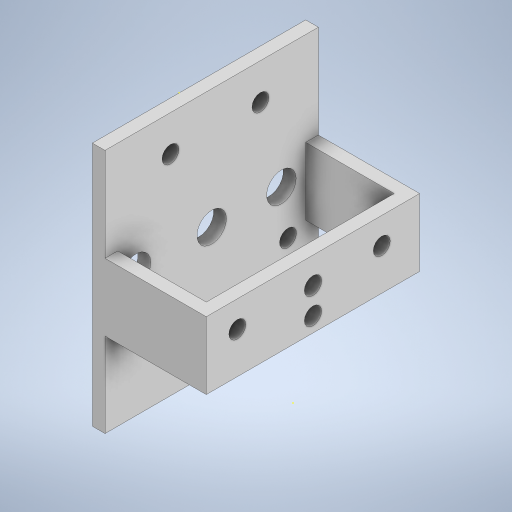
# Autodesk Inventor part: korthjulholder1
Saved by Autodesk Inventor 2023 (Build 270158000, 158)
## iProperties
Created: 2023-02-28
Part Number: korthjulholder1
Material: Generic
Document SubType Name: Modeling
Designer: Markus
Density: 1 g/cm^3
Appearance: Default
Author: Markus
Autodesk Inventor part; units mm, degrees
ref_plane "YZ Plane" through (0, 0, 0) normal (1, 0, 0) x (0, 1, 0)
ref_plane "XZ Plane" through (0, 0, 0) normal (0, 1, 0) x (-1, 0, 0)
ref_plane "XY Plane" through (0, 0, 0) normal (0, 0, 1) x (1, 0, 0)
sketch "Sketch1" plane through (0, 0, 0) normal (1, 0, 0) x (0, 1, 0)
  line L0 (0, 0) -> (20, 0)
  line L1 (20, 0) -> (20, -25)
  line L2 (20, -25) -> (0, -25)
  line L3 (0, -25) -> (0, 0)
  dimension "d0" = 20
  dimension "d1" = 25
  constraints: 8 end point, 2 parallel, 1 horizontal, 1 perpendicular
  measures "d0" distance of L1.end L2.end
  measures "d1" distance of L0.end L1.end
extrude "Extrusion1" add sketch "Sketch1" along normal blind 2
sketch "Sketch2" plane through (2, 0, 0) normal (1, 0, 0) x (0, 0, -1)
  line L0 (25, 0) -> (25, 20) projected
  line L1 (0, 0) -> (25, 0)
  line L2 (25, 0) -> (25, 2)
  line L3 (25, 2) -> (0, 2)
  line L4 (0, 2) -> (0, 0)
  dimension "d4" = 2
  constraints: 8 end point, 2 parallel, 1 horizontal, 1 perpendicular, 1 point on line
  measures "d4" distance of L2.end L1.end
extrude "Extrusion2" add sketch "Sketch2" along normal blind 25
sketch "Sketch3" plane through (2, 2, 0) normal (0, 1, 0) x (1, 0, 0)
  line L0 (-2, 0) -> (25, 0) projected
  line L1 (-2, 25) -> (25, 25) projected
  line L2 (25, 0) -> (23, 0)
  line L3 (23, 0) -> (23, 25)
  line L4 (23, 25) -> (25, 25)
  line L5 (25, 25) -> (25, 0)
  dimension "d7" = 2
  constraints: 8 end point, 2 parallel, 1 horizontal, 1 perpendicular, 1 point on line
  measures "d7" distance of L3.end L4.end
extrude "Extrusion3" add sketch "Sketch3" along normal blind 20
sketch "Sketch4" plane through (2, 0, 0) normal (1, 0, 0) x (0, 0, -1)
  point P0 (0, 0)
sketch "Sketch5" plane through (27, 0, 0) normal (1, 0, 0) x (0, 0, -1)
  circle A0 centre (6, 19.5) radius 2
  point P0 (0, 0)
  dimension "d10" = 4
  constraints: 1 centre point, 1 coincident
  measures "d10" diameter of A0
sketch "Sketch6" plane through (2, 22, 0) normal (0, 1, 0) x (1, 0, 0)
  line L0 (25, 0) -> (25, 25) projected
  line L1 (23, 25) -> (23, 0) projected
  line L2 (25, 0) -> (23, 0)
  line L3 (23, 0) -> (23, 25)
  line L4 (23, 25) -> (25, 25)
  line L5 (25, 25) -> (25, 0)
  point P0 (-2, 0)
  constraints: 8 end point, 2 parallel, 1 horizontal, 1 perpendicular
extrude "Extrusion4" add sketch "Sketch6" along normal blind 3
sketch "Sketch7" plane through (0, 20, 0) normal (0, 1, 0) x (1, 0, 0)
  line L0 (0, 25) -> (2, 25) projected
  line L1 (2, 25) -> (0, 25)
  line L2 (0, 25) -> (0, 0)
  line L3 (0, 0) -> (2, 0)
  line L4 (2, 0) -> (2, 25)
  constraints: 8 end point, 2 parallel, 1 horizontal, 1 perpendicular
extrude "Extrusion5" add sketch "Sketch7" along normal blind 5
extrude "Extrusion6" cut sketch "Sketch5" against normal blind 30
sketch "Sketch8" plane through (0, 0, 0) normal (-1, 0, 0) x (0, 0, 1)
  circle A0 centre (-22.8, 23) radius 2
  point P0 (0, 0)
  point P1 (22.8, 23)
  dimension "d17" = 4
  constraints: 1 centre point, 1 coincident
  measures "d17" diameter of A0
sketch "Sketch9" plane through (0, 0, 0) normal (-1, 0, 0) x (0, 0, 1)
  circle A0 centre (-6, 19.5) radius 2 projected
  circle A1 centre (-6, 19.5) radius 2
  point P0 (0, 0)
  constraints: 1 centre point, 1 coincident
extrude "Extrusion7" add sketch "Sketch9" against normal blind 2
extrude "Extrusion8" cut sketch "Sketch8" against normal blind 30
sketch "Sketch10" plane through (0, 0, -25) normal (-1, 0, 0) x (0, 0, 1)
  line L0 (25, 25) -> (2.2, 25) projected
  line L1 (25, 0) -> (0, 0) projected
  line L2 (12.5, 25) -> (25, 25)
  line L3 (25, 25) -> (25, 0)
  line L4 (25, 0) -> (12.5, 0)
  line L5 (12.5, 0) -> (12.5, 25)
  constraints: 8 end point, 2 parallel, 1 horizontal, 1 perpendicular, 1 point on line
extrude "Extrusion9" cut sketch "Sketch10" against normal blind 30
sketch "Sketch11" plane through (0, 0, -25) normal (-1, 0, 0) x (0, 0, 1)
  circle A0 centre (10.3, 23) radius 2
  point P0 (25, 0)
  dimension "d24" = 4
  constraints: 1 centre point, 1 coincident
  measures "d24" diameter of A0
extrude "Extrusion10" cut sketch "Sketch11" against normal blind 2.5
sketch "Sketch12" plane through (27, 0, -25) normal (1, 0, 0) x (0, 0, -1)
  circle A0 centre (-2.2, 23) radius 2 projected
  line L0 (-12.5, 25) -> (-10.3, 25) projected
  line L1 (-12.5, 2) -> (0, 2) projected
  line L2 (-12.5, 25) -> (-4.5, 25)
  line L3 (-4.5, 25) -> (-4.5, 2)
  line L4 (-4.5, 2) -> (-12.5, 2)
  line L5 (-12.5, 2) -> (-12.5, 25)
  point P0 (-25, 0)
  point P1 (-4.2, 23)
  point P2 (-2.2, 25)
  dimension "d27" = 8
  constraints: 8 end point, 2 parallel, 1 horizontal, 1 perpendicular, 1 point on circle, 1 point on line
  measures "d27" distance of L3.end L4.end
sketch "Sketch13" plane through (27, 0, -25) normal (1, 0, 0) x (0, 0, -1)
  point P0 (-25, 0)
sketch "Sketch14" plane through (0, 0, -25) normal (0, -1, 0) x (1, 0, 0)
  line L0 (27, 12.5) -> (0, 12.5) projected
  line L1 (25, 12.5) -> (25, 0) projected
  line L2 (27, 12.5) -> (25, 12.5)
  line L3 (25, 12.5) -> (25, 0)
  line L4 (25, 0) -> (27, 0)
  line L5 (27, 0) -> (27, 12.5)
  point P0 (0, 25)
  constraints: 8 end point, 2 parallel, 1 horizontal, 1 perpendicular
extrude "Extrusion11" add sketch "Sketch14" along normal blind 8
extrude "Extrusion12" cut sketch "Sketch12" against normal blind 8 contours L0 L2 L3 L1 L5
sketch "Sketch15" plane through (25, 2, -25) normal (0, 0, -1) x (-1, 0, 0)
  line L0 (0, -2) -> (0, -10) projected
  line L1 (0, -2) -> (25, -2)
  line L2 (25, -2) -> (25, 23)
  line L3 (25, 23) -> (0, 23)
  line L4 (0, 23) -> (0, -2)
  constraints: 8 end point, 2 parallel, 1 horizontal, 1 perpendicular
extrude "Extrusion13" cut sketch "Sketch15" against normal blind 30
sketch "Sketch16" plane through (27, 23, -22.8) normal (1, 0, 0) x (0, 0, -1)
  arc A0 (-0.0621, -1.999) -> (-0.0621, 1.999) centre (0, 0) ccw projected
  circle A1 centre (0, 0) radius 2
  point P0 (-22.8, -23)
  point P1 (0, 2)
  point P2 (-36, 0)
  point P3 (-0.0621, 1.999)
  point P4 (-0.0621, -1.999)
  dimension "d34" = 4
  constraints: 4 coincident, 1 centre point
  measures "d34" diameter of A1
sketch "Sketch17" plane through (25, 2, -12.5) normal (0, 0, 1) x (1, 0, 0)
  point P0 (-25, -2)
sketch "Sketch18" plane through (25, 2, -12.5) normal (0, 0, 1) x (1, 0, 0)
  line L0 (0, -10) -> (2, -10) projected
  line L1 (2, 0) -> (0, 0) projected
  line L2 (2, -10) -> (0, -10)
  line L3 (0, -10) -> (0, 0)
  line L4 (0, 0) -> (2, 0)
  line L5 (2, 0) -> (2, -10)
  point P0 (-25, -2)
  constraints: 8 end point, 2 parallel, 1 horizontal, 1 perpendicular
extrude "Extrusion14" add sketch "Sketch18" along normal blind 30
sketch "Sketch19" plane through (27, 23, -22.8) normal (1, 0, 0) x (0, 0, -1)
  point P0 (-22.8, -23)
sketch "Sketch20" plane through (25, 2, -20.5) normal (0, 1, 0) x (1, 0, 0)
  line L0 (2, 0) -> (2, 2.3) projected
  line L1 (0, 4.5) -> (0, -38) projected
  line L2 (2, 0) -> (0, 0)
  line L3 (0, 0) -> (0, -38)
  line L4 (0, -38) -> (2, -38)
  line L5 (2, -38) -> (2, 0)
  point P0 (-25, -20.5)
  constraints: 8 end point, 2 parallel, 1 horizontal, 1 perpendicular
extrude "Extrusion15" add sketch "Sketch20" along normal blind 23
sketch "Sketch21" plane through (27, 23, -22.8) normal (1, 0, 0) x (0, 0, -1)
  point P0 (-22.8, -23)
sketch "Sketch22" plane through (27, 23, -22.8) normal (1, 0, 0) x (0, 0, -1)
  point P0 (-22.8, -23)
sketch "Sketch23" plane through (27, 23, -22.8) normal (1, 0, 0) x (0, 0, -1)
  circle A0 centre (-36, 0) radius 2
  point P0 (-22.8, -23)
  dimension "d39" = 4
  constraints: 1 centre point, 1 coincident
  measures "d39" diameter of A0
extrude "Extrusion16" cut sketch "Sketch23" against normal blind 25
sketch "Sketch24" plane through (27, 23, -22.8) normal (1, 0, 0) x (0, 0, -1)
  circle A0 centre (-36, 0) radius 2 projected
  line L0 (-36, 2) -> (-40.3, 2) projected
  line L1 (2.2, -31) -> (-40.3, -31) projected
  line L2 (-40.3, 2) -> (-38.3, 2)
  line L3 (-38.3, 2) -> (-38.3, -31)
  line L4 (-38.3, -31) -> (-40.3, -31)
  line L5 (-40.3, -31) -> (-40.3, 2)
  point P0 (-22.8, -23)
  point P1 (-38, 0)
  dimension "d42" = 2
  constraints: 8 end point, 2 parallel, 1 horizontal, 1 perpendicular, 1 point on circle, 1 point on line
  measures "d42" distance of L3.end L4.end
extrude "Extrusion17" cut sketch "Sketch24" against normal blind 25 contours L3 L1 L5 L0
sketch "Sketch25" plane through (25, 23, -22.8) normal (-1, 0, 0) x (0, 0, 1)
  circle A0 centre (0, 0) radius 2 projected
  line L0 (36, 2) -> (0, 2) projected
  line L1 (2, 0) -> (2.3, 0)
  line L2 (2.3, 0) -> (2.3, 2)
  line L3 (2.3, 2) -> (2, 2)
  line L4 (2, 2) -> (2, 0)
  circle A1 centre (36, 0) radius 2 projected
  line L5 (34, 0) -> (33.7, 0)
  line L6 (33.7, 0) -> (33.7, 0.0469)
  line L7 (33.7, 0.0469) -> (34, 0.0469)
  line L8 (34, 0.0469) -> (34, 0)
  line L9 (2.3, 2) -> (33.7, 2)
  line L10 (33.7, 2) -> (33.7, 0)
  line L11 (33.7, 0) -> (2.3, 0)
  line L12 (2.3, 0) -> (2.3, 2)
  point P0 (22.8, -23)
  point P1 (2.3, 0)
  point P2 (33.7, 0.0469)
  dimension "d45" = 0.3
  dimension "d46" = 0.3
  constraints: 24 end point, 6 parallel, 3 horizontal, 3 perpendicular, 2 point on circle, 1 point on line
  measures "d45" distance of L3.end L2.end
  measures "d46" distance of L6.end L7.end
extrude "Extrusion18" cut sketch "Sketch25" against normal blind 25 contours L2 L0 L10 L6 L11
sketch "Sketch26" plane through (25, 23, -22.8) normal (-1, 0, 0) x (0, 0, 1)
  line L0 (-2.2, -31) -> (38.3, -31) projected
  line L1 (38.3, -31) -> (38.3, 2) projected
  line L2 (-2.2, -31) -> (38.3, -31)
  line L3 (38.3, -31) -> (38.3, -29)
  line L4 (38.3, -29) -> (-2.2, -29)
  line L5 (-2.2, -29) -> (-2.2, -31)
  line L6 (2.3, 0) -> (33.7, 0) projected
  line L7 (2.3, 0) -> (33.7, 0)
  line L8 (33.7, 0) -> (33.7, -29)
  line L9 (33.7, -29) -> (2.3, -29)
  line L10 (2.3, -29) -> (2.3, 0)
  point P0 (22.8, -23)
  dimension "d49" = 2
  constraints: 16 end point, 4 parallel, 2 horizontal, 2 perpendicular, 2 point on line
  measures "d49" distance of L3.end L2.end
extrude "Extrusion19" cut sketch "Sketch26" against normal blind 25 contours L10 L6 L8 L4
sketch "Sketch27" plane through (25, 23, -22.8) normal (-1, 0, 0) x (0, 0, 1)
  line L0 (-2.2, -31) -> (38.3, -31) projected
  line L1 (38.3, 2) -> (38.3, -31) projected
  line L2 (-2.2, -31) -> (38.3, -31)
  line L3 (38.3, -31) -> (38.3, -28.9821)
  line L4 (38.3, -28.9821) -> (-2.2, -28.9821)
  line L5 (-2.2, -28.9821) -> (-2.2, -31)
  point P0 (22.8, -23)
  constraints: 8 end point, 2 parallel, 1 horizontal, 1 perpendicular, 1 point on line
extrude "Extrusion20" add sketch "Sketch27" along normal blind 25
sketch "Sketch28" plane through (25, -5.9821, 10.9) normal (0, 1, 0) x (1, 0, 0)
  line L0 (2, -4.6) -> (-25, -4.6) projected
  line L1 (2, 35.9) -> (-25, 35.9) projected
  line L2 (-25, -4.6) -> (-22, -4.6)
  line L3 (-22, -4.6) -> (-22, 35.9)
  line L4 (-22, 35.9) -> (-25, 35.9)
  line L5 (-25, 35.9) -> (-25, -4.6)
  point P0 (-25, 10.9)
  dimension "d54" = 3
  constraints: 8 end point, 2 parallel, 1 horizontal, 1 perpendicular, 1 point on line
  measures "d54" distance of L4.end L3.end
extrude "Extrusion21" add sketch "Sketch28" along normal blind 31
sketch "Sketch29" plane through (27, -8, 15.5) normal (0, 0, 1) x (1, 0, 0)
  point P0 (-27, 8)
sketch "Sketch30" plane through (27, -8, 15.5) normal (0, 0, 1) x (1, 0, 0)
  line L0 (-27, 0) -> (-27, 33.0179) projected
  line L1 (-24, 2.0179) -> (-24, 33.0179) projected
  line L2 (-27, 33.0179) -> (-24, 33.0179)
  line L3 (-24, 33.0179) -> (-24, 32.9999)
  line L4 (-24, 32.9999) -> (-27, 32.9999)
  line L5 (-27, 32.9999) -> (-27, 33.0179)
  point P0 (-27, 8)
  dimension "d57" = 0.018
  constraints: 8 end point, 2 parallel, 1 horizontal, 1 perpendicular, 1 point on line
  measures "d57" distance of L2.end L3.end
extrude "Extrusion22" cut sketch "Sketch30" against normal blind 31
sketch "Sketch31" plane through (0, 23, -22.8) normal (-1, 0, 0) x (0, 0, 1)
  circle A0 centre (0, -12.5) radius 2
  point P0 (22.8, -23)
  point P1 (36, -12500)
  point P2 (36, -12500)
  dimension "d60" = 4
  constraints: 2 coincident, 1 centre point
  measures "d60" diameter of A0
sketch "Sketch32" plane through (0, 23, -22.8) normal (-1, 0, 0) x (0, 0, 1)
  circle A0 centre (36.1, -12.4998) radius 2
  point P0 (22.8, -23)
  point P1 (-0.0002, -12.4998)
  dimension "d61" = 4
  constraints: 1 centre point, 1 coincident
  measures "d61" diameter of A0
extrude "Extrusion23" cut sketch "Sketch31" against normal blind 3
extrude "Extrusion24" cut sketch "Sketch32" against normal blind 3
fillet "Fillet1" radius 2 2 edges at (1.5, 24.9999, 15.5) (1.5, 25.0179, -25)
fillet "Fillet2" radius 2 2 edges at (0, -8, -4.75) (27, -8, -4.75)
sketch "Sketch33" plane through (0, 23, -22.8) normal (-1, 0, 0) x (0, 0, 1)
  point P0 (22.8, -23)
sketch "Sketch34" plane through (0, 23, -22.8) normal (-1, 0, 0) x (0, 0, 1)
  circle A0 centre (18.05, -4) radius 2
  point P0 (22.8, -23)
  dimension "d68" = 4
  constraints: 1 centre point, 1 coincident
  measures "d68" diameter of A0
extrude "Extrusion25" cut sketch "Sketch34" against normal blind 3
sketch "Sketch35" plane through (27, 23, 13.2) normal (1, 0, 0) x (0, 0, -1)
  point P0 (13.2, -23)
sketch "Sketch36" plane through (25, -6, 10.9) normal (0, 1, 0) x (1, 0, 0)
  line L0 (0, 0) -> (2, 0) projected
  line L1 (0, 0) -> (0, 31.4) projected
  line L2 (2, 0) -> (0, 0)
  line L3 (0, 0) -> (0, 31.4)
  line L4 (0, 31.4) -> (2, 31.4)
  line L5 (2, 31.4) -> (2, 0)
  point P0 (-25, 10.9)
  constraints: 8 end point, 2 parallel, 1 horizontal, 1 perpendicular
extrude "Extrusion26" add sketch "Sketch36" along normal blind 3
sketch "Sketch37" plane through (27, 23, -22.8) normal (1, 0, 0) x (0, 0, -1)
  point P0 (-22.8, -23)
sketch "Sketch38" plane through (25, -3, 10.9) normal (0, 1, 0) x (1, 0, 0)
  line L0 (2, 0) -> (0, 0) projected
  line L1 (2, 35.9) -> (2, -4.6) projected
  line L2 (0, 0) -> (2, 0)
  line L3 (2, 0) -> (2, 31.4499)
  line L4 (2, 31.4499) -> (0, 31.4499)
  line L5 (0, 31.4499) -> (0, 0)
  point P0 (-25, 10.9)
  constraints: 8 end point, 2 parallel, 1 horizontal, 1 perpendicular, 1 point on line
extrude "Extrusion27" add sketch "Sketch38" along normal blind 3
sketch "Sketch39" plane through (25, 0, 10.9) normal (0, 1, 0) x (1, 0, 0)
  line L0 (0, 31.4) -> (0, 0) projected
  line L1 (2, 0) -> (2, 31.4) projected
  line L2 (0, 0) -> (2, 0)
  line L3 (2, 0) -> (2, 31.4)
  line L4 (2, 31.4) -> (0, 31.4)
  line L5 (0, 31.4) -> (0, 0)
  point P0 (-25, 10.9)
  constraints: 8 end point, 2 parallel, 1 horizontal, 1 perpendicular
extrude "Extrusion28" add sketch "Sketch39" along normal blind 25
sketch "Sketch40" plane through (27, 23, -22.8) normal (1, 0, 0) x (0, 0, -1)
  point P0 (-22.8, -23)
sketch "Sketch41" plane through (2, 25, 0) normal (0, 1, 0) x (1, 0, 0)
  line L0 (25, -15.5) -> (23, -15.5) projected
  line L1 (25, 22.8) -> (25, 25) projected
  line L2 (23, -15.5) -> (25, -15.5)
  line L3 (25, -15.5) -> (25, 25)
  line L4 (25, 25) -> (23, 25)
  line L5 (23, 25) -> (23, -15.5)
  point P0 (-2, 0)
  constraints: 8 end point, 2 parallel, 1 horizontal, 1 perpendicular
extrude "Extrusion29" add sketch "Sketch41" along normal blind 3
sketch "Sketch42" plane through (3, -5.9821, 15.5) normal (0, 0, 1) x (1, 0, 0)
  line L0 (22, 0) -> (0, 0) projected
  line L1 (24, 33.9821) -> (24, -0.0179) projected
  line L2 (22, 0) -> (24, 0)
  line L3 (24, 0) -> (24, 33.9821)
  line L4 (24, 33.9821) -> (22, 33.9821)
  line L5 (22, 33.9821) -> (22, 0)
  point P0 (-3, 5.9821)
  constraints: 8 end point, 2 parallel, 1 horizontal, 1 perpendicular
extrude "Extrusion30" add sketch "Sketch42" along normal blind 5
sketch "Sketch43" plane through (25, -5.9821, -25) normal (0, 0, -1) x (-1, 0, 0)
  arc A0 (-2, -0.0179) -> (0, -2.0179) centre (0, -0.0179) ccw projected
  line L0 (0, 33.9821) -> (0, 0) projected
  line L1 (-2, -0.0179) -> (0, -0.0179)
  line L2 (0, -0.0179) -> (0, 33.9821)
  line L3 (0, 33.9821) -> (-2, 33.9821)
  line L4 (-2, 33.9821) -> (-2, -0.0179)
  point P0 (25, 5.9821)
  constraints: 8 end point, 2 parallel, 1 horizontal, 1 perpendicular
extrude "Extrusion31" add sketch "Sketch43" along normal blind 5
sketch "Sketch44" plane through (25, -5.9821, -25) normal (0, 0, -1) x (-1, 0, 0)
  point P0 (25, 5.9821)
sketch "Sketch45" plane through (0, -8, -25) normal (0, -1, 0) x (1, 0, 0)
  point P0 (0, 25)
sketch "Sketch46" plane through (0, -8, -25) normal (0, -1, 0) x (1, 0, 0)
  line L0 (27, 40.5) -> (0, 40.5)
  line L1 (0, 40.5) -> (0, 0)
  line L2 (0, 0) -> (27, 0)
  line L3 (27, 0) -> (27, 40.5)
  point P0 (0, 25)
  constraints: 8 end point, 2 parallel, 1 horizontal, 1 perpendicular
extrude "Extrusion32" cut sketch "Sketch46" against normal up to surface (2.0179 mm away)
sketch "Sketch47" plane through (27, 0, 0) normal (1, 0, 0) x (0, 0, -1)
  point P0 (0, 0)
sketch "Sketch48" plane through (25, -5.9821, 20.5) normal (0, -1, 0) x (1, 0, 0)
  line L0 (2, -50.5) -> (0, -50.5) projected
  line L1 (2, -50.5) -> (-25, -50.5)
  line L2 (-25, -50.5) -> (-25, 0.0671)
  line L3 (-25, 0.0671) -> (2, 0.0671)
  line L4 (2, 0.0671) -> (2, -50.5)
  point P0 (-25, -20.5)
  constraints: 8 end point, 2 parallel, 1 horizontal, 1 perpendicular
extrude "Extrusion33" add sketch "Sketch48" along normal blind 2
sketch "Sketch49" plane through (0, 23, -22.8) normal (-1, 0, 0) x (0, 0, 1)
  line L0 (-2.2, -28.9821) -> (-2.2, 0.0179) projected
  line L1 (-2.2, 0.0179) -> (38.3, 0.0179)
  line L2 (38.3, 0.0179) -> (38.3, 1.9999)
  line L3 (38.3, 1.9999) -> (-2.2, 1.9999)
  line L4 (-2.2, 1.9999) -> (-2.2, 0.0179)
  point P0 (22.8, -23)
  constraints: 8 end point, 2 parallel, 1 horizontal, 1 perpendicular
extrude "Extrusion34" cut sketch "Sketch49" against normal blind 5
sketch "Sketch50" plane through (0, 23, -22.8) normal (-1, 0, 0) x (0, 0, 1)
  line L0 (7.3, 1.9999) -> (-0.4677, 1.9999) projected
  line L1 (-0.4677, 1.9999) -> (7.3, 1.9999)
  line L2 (7.3, 1.9999) -> (7.3, 2.0583)
  line L3 (7.3, 2.0583) -> (-0.4677, 2.0583)
  line L4 (-0.4677, 2.0583) -> (-0.4677, 1.9999)
  point P0 (22.8, -23)
  constraints: 8 end point, 2 parallel, 1 horizontal, 1 perpendicular
extrude "Extrusion35" cut sketch "Sketch50" against normal blind 5
sketch "Sketch51" plane through (25, -5.9821, 20.5) normal (0, 1, 0) x (1, 0, 0)
  line L0 (-25, 45.5) -> (-25, 50.5) projected
  line L1 (-22, 45.5) -> (-25, 45.5) projected
  line L2 (-25, 50.5) -> (-22, 50.5)
  line L3 (-22, 50.5) -> (-22, 45.5)
  line L4 (-22, 45.5) -> (-25, 45.5)
  line L5 (-25, 45.5) -> (-25, 50.5)
  line L6 (-25, 5) -> (-22, 5) projected
  line L7 (-25, -0.0671) -> (-25, 5) projected
  line L8 (-22, 5) -> (-25, 5)
  line L9 (-25, 5) -> (-25, -0.0671)
  line L10 (-25, -0.0671) -> (-22, -0.0671)
  line L11 (-22, -0.0671) -> (-22, 5)
  point P0 (-25, 20.5)
  constraints: 16 end point, 4 parallel, 2 horizontal, 2 perpendicular
extrude "Extrusion36" add sketch "Sketch51" along normal up to surface (29 mm away)
sketch "Sketch52" plane through (0, 23.0179, 15.4999) normal (0, 1, 0) x (1, 0, 0)
  line L0 (3, 0) -> (3, 45.4999) projected
  line L1 (0, -0.0001) -> (0, -5.0672) projected
  line L2 (3, 45.4999) -> (0, 45.4999)
  line L3 (0, 45.4999) -> (0, -5.0672)
  line L4 (0, -5.0672) -> (3, -5.0672)
  line L5 (3, -5.0672) -> (3, 45.4999)
  point P0 (0, 15.4999)
  constraints: 8 end point, 2 parallel, 1 horizontal, 1 perpendicular
extrude "Extrusion37" add sketch "Sketch52" along normal blind 50
sketch "Sketch53" plane through (0, 23, -22.8) normal (-1, 0, 0) x (0, 0, 1)
  circle A0 centre (18.05, -4) radius 2 projected
  circle A1 centre (0, -12.5) radius 2 projected
  circle A2 centre (36.1, -12.4998) radius 2 projected
  circle A3 centre (0, 38.0418) radius 2
  circle A4 centre (18.05, 38.0418) radius 2
  circle A5 centre (36.1, 38.0418) radius 2
  circle A6 centre (18.05, -4) radius 2
  point P0 (22.8, -23)
  dimension "d95" = 4
  dimension "d96" = 4
  dimension "d97" = 4
  constraints: 7 coincident, 4 centre point, 1 concentric
  measures "d95" diameter of A3
  measures "d96" diameter of A4
  measures "d97" diameter of A5
extrude "Extrusion38" cut sketch "Sketch53" against normal blind 50 contours A3 | A4 | A5
sketch "Sketch54" plane through (0, 23, -22.8) normal (-1, 0, 0) x (0, 0, 1)
  circle A0 centre (18.05, -4) radius 2 projected
  circle A1 centre (18.05, -4) radius 2
  point P0 (22.8, -23)
  constraints: 2 coincident, 1 centre point, 1 concentric
extrude "Extrusion39" add sketch "Sketch54" against normal blind 3
sketch "Sketch55" plane through (25, -5.9821, 20.5) normal (0, 1, 0) x (1, 0, 0)
  line L0 (0, 50.5) -> (2, 50.5) projected
  line L1 (2, -0.0671) -> (-22, -0.0671) projected
  line L2 (0, 50.5) -> (-1, 50.5)
  line L3 (-1, 50.5) -> (-1, -0.0671)
  line L4 (-1, -0.0671) -> (0, -0.0671)
  line L5 (0, -0.0671) -> (0, 50.5)
  point P0 (-25, 20.5)
  point P1 (0, -0.0671)
  dimension "d102" = 1
  constraints: 8 end point, 2 parallel, 1 horizontal, 1 perpendicular, 1 point on line
  measures "d102" distance of L4.end L3.end
extrude "Extrusion40" add sketch "Sketch55" along normal up to surface (33.9821 mm away)
sketch "Sketch56" plane through (25, -5.9821, 20.5) normal (0, 1, 0) x (1, 0, 0)
  line L0 (-22, 50.5) -> (-1, 50.5) projected
  line L1 (0, -0.0671) -> (-1, -0.0671) projected
  line L2 (-22, 50.5) -> (-1, 50.5)
  line L3 (-1, 50.5) -> (-1, -0.0671)
  line L4 (-1, -0.0671) -> (-22, -0.0671)
  line L5 (-22, -0.0671) -> (-22, 50.5)
  point P0 (-25, 20.5)
  constraints: 8 end point, 2 parallel, 1 horizontal, 1 perpendicular
extrude "Extrusion41" add sketch "Sketch56" along normal blind 1
sketch "Sketch57" plane through (3, -5.9821, 20.5) normal (0, 0, 1) x (1, 0, 0)
  line L0 (22, 0) -> (22, 33.9821) projected
  line L1 (24, 33.9821) -> (24, -2) projected
  line L2 (22, 33.9821) -> (24, 33.9821)
  line L3 (24, 33.9821) -> (24, -0.0257)
  line L4 (24, -0.0257) -> (22, -0.0257)
  line L5 (22, -0.0257) -> (22, 33.9821)
  point P0 (-3, 5.9821)
  constraints: 8 end point, 2 parallel, 1 horizontal, 1 perpendicular, 1 point on line
extrude "Extrusion42" add sketch "Sketch57" along normal up to surface (0.0671 mm away)
sketch "Sketch58" plane through (27, 0, 0) normal (1, 0, 0) x (0, 0, -1)
  point P0 (0, 0)
sketch "Sketch59" plane through (25, 23, 13.2) normal (1, 0, 0) x (0, 0, -1)
  circle A0 centre (0, 0) radius 1.9931
  circle A1 centre (36.0442, 0) radius 2.0019
  point P0 (13.2, -23)
  constraints: 2 centre point, 1 coincident
extrude "Extrusion43" cut sketch "Sketch59" against normal blind 10
sketch "Sketch60" plane through (27, 0, 0) normal (1, 0, 0) x (0, 0, -1)
  circle A0 centre (4.75, 61.0418) radius 2 projected
  line L0 (-1.2836, 17.728) -> (10.7164, 17.728)
  line L1 (10.7164, 17.728) -> (10.7164, 28)
  line L2 (10.7164, 28) -> (-1.2836, 28)
  line L3 (-1.2836, 28) -> (-1.2836, 17.728)
  line L4 (-1.2836, 17.728) -> (10.7164, 28) construction
  line L5 (10.7164, 17.728) -> (-1.2836, 28) construction
  line L6 (-1.2836, 22.864) -> (10.7164, 22.864)
  line L7 (10.7164, 22.864) -> (10.7164, 28)
  line L8 (10.7164, 28) -> (-1.2836, 28)
  line L9 (-1.2836, 28) -> (-1.2836, 22.864)
  point P0 (0, 0)
  point P1 (4.7164, 22.864)
  dimension "d111" = 12
  constraints: 20 end point, 4 parallel, 3 midpoint, 2 horizontal, 2 perpendicular, 1 coincident
  measures "d111" distance of L0.start L0.end
extrude "Extrusion44" cut sketch "Sketch60" against normal blind 10 contours L3 L2 L1 L6
fillet "Fillet3" radius 2 2 edges at (25.5, 28, 1.2836) (25.5, 28, -10.7164)
sketch "Sketch61" plane through (27, 0, 0) normal (1, 0, 0) x (0, 0, -1)
  line L0 (-1.2836, 22.864) -> (10.7164, 22.864)
  line L1 (10.7164, 22.864) -> (10.7164, 18.864)
  line L2 (10.7164, 18.864) -> (-1.2836, 18.864)
  line L3 (-1.2836, 18.864) -> (-1.2836, 22.864)
  point P0 (0, 0)
  dimension "d115" = 4
  constraints: 8 end point, 2 parallel, 1 horizontal, 1 perpendicular
  measures "d115" distance of L0.end L1.end
extrude "Extrusion45" cut sketch "Sketch61" against normal blind 10
sketch "Sketch62" plane through (25, -7.9821, 20.5) normal (0, -1, 0) x (1, 0, 0)
  point P0 (-25, -20.5)
sketch "Sketch63" plane through (27, 0, 0) normal (1, 0, 0) x (0, 0, -1)
  line L0 (-1.2836, 18.864) -> (10.7164, 18.864) projected
  line L1 (12.7164, 28) -> (30, 28) projected
  line L2 (10.7164, 18.864) -> (16.2164, 18.864)
  line L3 (16.2164, 18.864) -> (16.2164, 28)
  line L4 (16.2164, 28) -> (10.7164, 28)
  line L5 (10.7164, 28) -> (10.7164, 18.864)
  line L6 (-1.2836, 26) -> (-1.2836, 18.864) projected
  line L7 (-20.5671, 28) -> (-3.2836, 28) projected
  line L8 (-1.2836, 18.864) -> (-6.7836, 18.864)
  line L9 (-6.7836, 18.864) -> (-6.7836, 28)
  line L10 (-6.7836, 28) -> (-1.2836, 28)
  line L11 (-1.2836, 28) -> (-1.2836, 18.864)
  point P0 (0, 0)
  dimension "d118" = 5.5
  dimension "d119" = 5.5
  constraints: 16 end point, 4 parallel, 2 horizontal, 2 perpendicular, 2 point on line
  measures "d118" distance of L4.end L3.end
  measures "d119" distance of L9.end L10.end
extrude "Extrusion46" cut sketch "Sketch63" against normal blind 10
sketch "Sketch64" plane through (25, -4.9821, 20.5) normal (0, 1, 0) x (1, 0, 0)
  line L0 (-25, -0.0671) -> (-22, -0.0671) projected
  line L1 (-1, 50.5) -> (-1, -0.0671) projected
  line L2 (-22, -0.0671) -> (-1, -0.0671)
  line L3 (-1, -0.0671) -> (-1, 2.9329)
  line L4 (-1, 2.9329) -> (-22, 2.9329)
  line L5 (-22, 2.9329) -> (-22, -0.0671)
  line L6 (-1, 50.5) -> (-22, 50.5) projected
  line L7 (-22, 50.5) -> (-1, 50.5)
  line L8 (-1, 50.5) -> (-1, 47.5)
  line L9 (-1, 47.5) -> (-22, 47.5)
  line L10 (-22, 47.5) -> (-22, 50.5)
  point P0 (-25, 20.5)
  point P1 (-1, 47.5)
  dimension "d122" = 3
  dimension "d123" = 3
  constraints: 16 end point, 4 parallel, 2 horizontal, 2 perpendicular, 2 point on line
  measures "d122" distance of L3.end L2.end
  measures "d123" distance of L7.end L8.end
extrude "Extrusion47" add sketch "Sketch64" along normal up to surface (32.9821 mm away)
sketch "Sketch65" plane through (0, -7.9821, 20.5671) normal (0, 0, 1) x (1, 0, 0)
  line L0 (3, 3) -> (24, 3) projected
  line L1 (24, 3) -> (24, 35.9821) projected
  line L2 (3, 3) -> (24, 3)
  line L3 (24, 3) -> (24, 9.5)
  line L4 (24, 9.5) -> (3, 9.5)
  line L5 (3, 9.5) -> (3, 3)
  point P0 (0, 7.9821)
  dimension "d126" = 6.5
  constraints: 8 end point, 2 parallel, 1 horizontal, 1 perpendicular, 1 point on line
  measures "d126" distance of L3.end L2.end
extrude "Extrusion48" cut sketch "Sketch65" against normal blind 70
fillet "Fillet4" radius 2 2 edges at (25.5, 28, 6.7836) (25.5, 28, -16.2164)
fillet "Fillet5" radius 2 2 edges at (1.5, 73.0179, -30) (1.5, 73.0179, 20.5671)
sketch "Sketch66" plane through (27, 0, 0) normal (1, 0, 0) x (0, 0, -1)
  line L0 (-8.7836, 28) -> (18.2164, 28)
  line L1 (18.2164, 28) -> (18.2164, 15.9597)
  line L2 (18.2164, 15.9597) -> (-8.7836, 15.9597)
  line L3 (-8.7836, 15.9597) -> (-8.7836, 28)
  point P0 (0, 0)
  constraints: 8 end point, 2 parallel, 1 horizontal, 1 perpendicular
extrude "Extrusion49" cut sketch "Sketch66" against normal blind 10
sketch "Sketch67" plane through (27, 0, 0) normal (1, 0, 0) x (0, 0, -1)
  point P0 (0, 0)
sketch "Sketch68" plane through (27, 0, 0) normal (1, 0, 0) x (0, 0, -1)
  point P0 (0, 0)
sketch "Sketch69" plane through (27, 0, 0) normal (1, 0, 0) x (0, 0, -1)
  point P0 (0, 0)
fillet "Fillet6" radius 2 2 edges at (25.5, 28, 8.7836) (25.5, 28, -18.2164)
sketch "Sketch70" plane through (0, 23, -22.8) normal (-1, 0, 0) x (0, 0, 1)
  line L0 (-7.2, 50.0179) -> (43.5303, 50.0179)
  line L1 (43.5303, 50.0179) -> (43.5303, 46.0179)
  line L2 (43.5303, 46.0179) -> (-7.2, 46.0179)
  line L3 (-7.2, 46.0179) -> (-7.2, 50.0179)
  point P0 (22.8, -23)
  dimension "d134" = 4
  constraints: 8 end point, 2 parallel, 1 horizontal, 1 perpendicular
  measures "d134" distance of L0.end L1.end
extrude "Extrusion50" add sketch "Sketch70" along normal blind 19
sketch "Sketch71" plane through (-19, 23, -22.8) normal (-1, 0, 0) x (0, 0, 1)
  line L0 (-5.2, 50.0179) -> (-7.2, 50.0179) projected
  line L1 (43.3671, 48.0179) -> (43.3671, 46.0179) projected
  line L2 (-7.2, 50.0179) -> (43.3671, 50.0179)
  line L3 (43.3671, 50.0179) -> (43.3671, 46.0179)
  line L4 (43.3671, 46.0179) -> (-7.2, 46.0179)
  line L5 (-7.2, 46.0179) -> (-7.2, 50.0179)
  point P0 (22.8, -23)
  constraints: 8 end point, 2 parallel, 1 horizontal, 1 perpendicular
extrude "Extrusion51" add sketch "Sketch71" along normal blind 3
sketch "Sketch72" plane through (0, 69.0179, -30) normal (0, -1, 0) x (1, 0, 0)
  line L0 (-19, 50.5671) -> (-22, 50.5671) projected
  line L1 (0, 0) -> (-22, 0) projected
  line L2 (-22, 50.5671) -> (-18.2142, 50.5671)
  line L3 (-18.2142, 50.5671) -> (-18.2142, 0)
  line L4 (-18.2142, 0) -> (-22, 0)
  line L5 (-22, 0) -> (-22, 50.5671)
  point P0 (0, 30)
  constraints: 8 end point, 2 parallel, 1 horizontal, 1 perpendicular, 1 point on line
extrude "Extrusion52" add sketch "Sketch72" along normal blind 20
fillet "Fillet7" radius 2 5 edges at (-9.5, 73.0179, 20.7303) (-11, 73.0179, -30) (-22, 73.0179, -4.7164) (-22, 61.0179, 20.5671) (-22, 61.0179, -30)
sketch "Sketch73" plane through (3, -4.9821, 20.5671) normal (1, 0, 0) x (0, 0, -1)
  line L0 (0, 74) -> (0, -3) projected
  line L1 (50.5671, 54) -> (0, 54) projected
  line L2 (0, 33.122) -> (50.5671, 33.122)
  line L3 (50.5671, 33.122) -> (50.5671, 54)
  line L4 (50.5671, 54) -> (0, 54)
  line L5 (0, 54) -> (0, 33.122)
  point P0 (20.5671, 4.9821)
  constraints: 8 end point, 2 parallel, 1 horizontal, 1 perpendicular, 1 point on line
extrude "Extrusion53" cut sketch "Sketch73" against normal blind 10
sketch "Sketch74" plane through (3, 73.0179, 18.5671) normal (1, 0, 0) x (0, 0, -1)
  point P0 (18.5671, -73.0179)
sketch "Sketch75" plane through (3, 73.0179, 18.5671) normal (1, 0, 0) x (0, 0, -1)
  line L0 (48.5671, -24) -> (-2, -24) projected
  line L1 (-2, -24) -> (48.5671, -24)
  line L2 (48.5671, -24) -> (48.5671, 2.4368)
  line L3 (48.5671, 2.4368) -> (-2, 2.4368)
  line L4 (-2, 2.4368) -> (-2, -24)
  point P0 (18.5671, -73.0179)
  constraints: 8 end point, 2 parallel, 1 horizontal, 1 perpendicular
extrude "Extrusion54" cut sketch "Sketch75" against normal blind 40
sketch "Sketch76" plane through (-19, 69.0179, 20.7303) normal (0, 0, 1) x (1, 0, 0)
  line L0 (-12.4602, -22.1181) -> (25.8897, -22.1181)
  line L1 (25.8897, -22.1181) -> (25.8897, 34.1617)
  line L2 (25.8897, 34.1617) -> (-12.4602, 34.1617)
  line L3 (-12.4602, 34.1617) -> (-12.4602, -22.1181)
  point P0 (19, -69.0179)
  constraints: 8 end point, 2 parallel, 1 horizontal, 1 perpendicular
extrude "Extrusion55" cut sketch "Sketch76" against normal blind 40
sketch "Sketch77" plane through (3, 28.1399, 20.5671) normal (0, 1, 0) x (1, 0, 0)
  line L0 (-3, 0) -> (-3, 50.5671) projected
  line L1 (0, 0) -> (0, 3) projected
  line L2 (-3, 50.5671) -> (0, 50.5671)
  line L3 (0, 50.5671) -> (0, 0)
  line L4 (0, 0) -> (-3, 0)
  line L5 (-3, 0) -> (-3, 50.5671)
  point P0 (-3, 20.5671)
  constraints: 8 end point, 2 parallel, 1 horizontal, 1 perpendicular
extrude "Extrusion56" add sketch "Sketch77" along normal blind 22
sketch "Sketch78" plane through (0, 23, -22.8) normal (-1, 0, 0) x (0, 0, 1)
  line L0 (43.3671, 27.1399) -> (-7.2, 27.1399) projected
  line L1 (-7.2, 27.1399) -> (44.6312, 27.1399)
  line L2 (44.6312, 27.1399) -> (44.6312, 24.1399)
  line L3 (44.6312, 24.1399) -> (-7.2, 24.1399)
  line L4 (-7.2, 24.1399) -> (-7.2, 27.1399)
  point P0 (22.8, -23)
  dimension "d150" = 3
  constraints: 8 end point, 2 parallel, 1 horizontal, 1 perpendicular
  measures "d150" distance of L1.end L2.end
extrude "Extrusion57" add sketch "Sketch78" along normal blind 21
sketch "Sketch79" plane through (0, 47.1399, -30) normal (0, -1, 0) x (1, 0, 0)
  line L0 (0, 0) -> (-21, 0) projected
  line L1 (0, 51.8312) -> (-21, 51.8312) projected
  line L2 (-21, 0) -> (-18, 0)
  line L3 (-18, 0) -> (-18, 51.8312)
  line L4 (-18, 51.8312) -> (-21, 51.8312)
  line L5 (-21, 51.8312) -> (-21, 0)
  point P0 (0, 30)
  dimension "d153" = 3
  constraints: 8 end point, 2 parallel, 1 horizontal, 1 perpendicular, 1 point on line
  measures "d153" distance of L4.end L3.end
extrude "Extrusion58" add sketch "Sketch79" along normal blind 21
sketch "Sketch80" plane through (0, 47.1399, 21.8312) normal (0, 0, 1) x (1, 0, 0)
  line L0 (-21, 3) -> (-21, -21) projected
  line L1 (3, 3) -> (-21, 3) projected
  line L2 (-21, -21) -> (0, -21)
  line L3 (0, -21) -> (0, 3)
  line L4 (0, 3) -> (-21, 3)
  line L5 (-21, 3) -> (-21, -21)
  point P0 (0, -47.1399)
  constraints: 8 end point, 2 parallel, 1 horizontal, 1 perpendicular, 1 point on line
extrude "Extrusion59" cut sketch "Sketch80" against normal up to surface (1.2641 mm away)
sketch "Sketch81" plane through (-21, 23, -22.8) normal (-1, 0, 0) x (0, 0, 1)
  circle A0 centre (36.1, -12.4998) radius 2 projected
  circle A1 centre (0.0369, 9.7943) radius 2
  circle A2 centre (36.1, 9.7943) radius 2
  point P0 (22.8, -23)
  dimension "d158" = 4
  dimension "d159" = 4
  constraints: 3 coincident, 2 centre point
  measures "d158" diameter of A1
  measures "d159" diameter of A2
extrude "Extrusion60" cut sketch "Sketch81" against normal blind 4 contours A1 | A2
sketch "Sketch82" plane through (-21, 23, -22.8) normal (-1, 0, 0) x (0, 0, 1)
  circle A0 centre (18.0836, 17.9735) radius 2
  point P0 (22.8, -23)
  dimension "d162" = 4
  constraints: 1 centre point
  measures "d162" diameter of A0
extrude "Extrusion61" cut sketch "Sketch82" against normal blind 4
sketch "Sketch83" plane through (27, 0, 0) normal (1, 0, 0) x (0, 0, -1)
  line L0 (-20.5671, 28) -> (-20.5671, -7.9821) projected
  line L1 (30, 28) -> (30, -7.9821) projected
  line L2 (-20.5671, 28) -> (30, 28)
  line L3 (30, 28) -> (30, 15.653)
  line L4 (30, 15.653) -> (-20.5671, 15.653)
  line L5 (-20.5671, 15.653) -> (-20.5671, 28)
  point P0 (0, 0)
  constraints: 8 end point, 2 parallel, 1 horizontal, 1 perpendicular, 1 point on line
extrude "Extrusion62" cut sketch "Sketch83" against normal up to surface (3 mm away)
sketch "Sketch84" plane through (27, 15.653, 20.5671) normal (0, 1, 0) x (1, 0, 0)
  line L0 (0, 50.5671) -> (0, 0) projected
  line L1 (-3, 0) -> (-3, 50.5671) projected
  line L2 (0, 50.5671) -> (-3, 50.5671)
  line L3 (-3, 50.5671) -> (-3, 0)
  line L4 (-3, 0) -> (0, 0)
  line L5 (0, 0) -> (0, 50.5671)
  point P0 (-27, 20.5671)
  constraints: 8 end point, 2 parallel, 1 horizontal, 1 perpendicular
extrude "Extrusion63" add sketch "Sketch84" along normal up to surface (12.347 mm away)
sketch "Sketch85" plane through (3, 50.1399, 20.5671) normal (0, 1, 0) x (1, 0, 0)
  point P0 (-3, 20.5671)
sketch "Sketch86" plane through (27, 0, 0) normal (1, 0, 0) x (0, 0, -1)
  line L0 (30, -7.9821) -> (-20.5671, -7.9821) projected
  circle A0 centre (4.7164, 21.7437) radius 2.05
  point P0 (0, 0)
  point P1 (4.7164, -7.9821)
  point P2 (-13.3386, 21.7437)
  point P3 (18.8202, 21.7437)
  dimension "d169" = 4.1
  constraints: 1 centre point, 1 coincident, 1 midpoint
  measures "d169" diameter of A0
extrude "Extrusion64" cut sketch "Sketch86" against normal blind 50
sketch "Sketch87" plane through (27, 0, 0) normal (1, 0, 0) x (0, 0, -1)
  circle A0 centre (4.7164, 21.7437) radius 2.05 projected
  circle A1 centre (-13.2168, 21.7437) radius 2
  circle A2 centre (21.0128, 21.7437) radius 2
  point P0 (0, 0)
  dimension "d172" = 4
  dimension "d173" = 4
  constraints: 3 coincident, 2 centre point
  measures "d172" diameter of A1
  measures "d173" diameter of A2
extrude "Extrusion65" cut sketch "Sketch87" against normal blind 50 contours A1 | A2
sketch "Sketch88" plane through (0, 23, -22.8) normal (-1, 0, 0) x (0, 0, 1)
  circle A0 centre (18.0836, -1.2563) radius 2.05 projected
  circle A1 centre (18.0836, -1.2563) radius 3.5
  circle A2 centre (36.0168, -1.2563) radius 2 projected
  circle A3 centre (36.0168, -1.2563) radius 3.5
  circle A4 centre (1.5719, -1.2563) radius 3.5
  point P0 (22.8, -23)
  dimension "d176" = 7
  dimension "d177" = 7
  dimension "d178" = 7
  constraints: 3 centre point, 2 coincident
  measures "d176" diameter of A1
  measures "d177" diameter of A3
  measures "d178" diameter of A4
extrude "Extrusion66" cut sketch "Sketch88" against normal blind 10 contours A0 | A1 | A2 | A3 | A4
sketch "Sketch89" plane through (-21, 23, -22.8) normal (-1, 0, 0) x (0, 0, 1)
  line L0 (-7.2, 3.1399) -> (43.3671, 3.1399) projected
  line L1 (43.3671, 27.1399) -> (-7.2, 27.1399) projected
  line L2 (-7.2, 3.1399) -> (43.3671, 3.1399)
  line L3 (43.3671, 3.1399) -> (43.3671, 27.1399)
  line L4 (43.3671, 27.1399) -> (-7.2, 27.1399)
  line L5 (-7.2, 27.1399) -> (-7.2, 3.1399)
  point P0 (22.8, -23)
  constraints: 8 end point, 2 parallel, 1 horizontal, 1 perpendicular
extrude "Extrusion67" cut sketch "Sketch89" against normal up to surface (21 mm away)
sketch "Sketch90" plane through (3, -4.9821, 20.5671) normal (1, 0, 0) x (0, 0, -1)
  circle A0 centre (15.5118, 46.5814) radius 2
  circle A1 centre (36.8292, 46.5814) radius 2
  point P0 (20.5671, 4.9821)
  dimension "d183" = 4
  dimension "d184" = 4
  constraints: 2 centre point
  measures "d183" diameter of A0
  measures "d184" diameter of A1
extrude "Extrusion68" cut sketch "Sketch90" against normal blind 10
sketch "Sketch91" plane through (27, 0, 0) normal (1, 0, 0) x (0, 0, -1)
  line L0 (-20.5671, -7.9821) -> (30, -7.9821) projected
  line L1 (30, 50.1399) -> (30, -7.9821) projected
  line L2 (-20.5671, -7.9821) -> (30, -7.9821)
  line L3 (30, -7.9821) -> (30, 12.0179)
  line L4 (30, 12.0179) -> (-20.5671, 12.0179)
  line L5 (-20.5671, 12.0179) -> (-20.5671, -7.9821)
  point P0 (0, 0)
  dimension "d187" = 20
  constraints: 8 end point, 2 parallel, 1 horizontal, 1 perpendicular, 1 point on line
  measures "d187" distance of L3.end L2.end
extrude "Extrusion69" cut sketch "Sketch91" against normal up to surface (24 mm away)
extrude "Extrusion70" add sketch "Sketch16" along normal blind 10
sketch "Sketch92" plane through (37, 23, -22.8) normal (1, 0, 0) x (0, 0, -1)
  circle A0 centre (0, 0) radius 2.3013
  point P0 (-22.8, -23)
  constraints: 1 centre point
extrude "Extrusion71" cut sketch "Sketch92" against normal up to surface (10 mm away)
sketch "Sketch93" plane through (3, -7.9821, 20.5671) normal (1, 0, 0) x (0, 0, -1)
  point P0 (20.5671, 7.9821)
sketch "Sketch94" plane through (3, -7.9821, 20.5671) normal (1, 0, 0) x (0, 0, -1)
  circle A0 centre (36.7074, 7.9821) radius 2
  circle A1 centre (16.4864, 7.9821) radius 2
  point P0 (20.5671, 7.9821)
  dimension "d194" = 4
  dimension "d195" = 4
  constraints: 2 centre point
  measures "d194" diameter of A0
  measures "d195" diameter of A1
extrude "Extrusion72" cut sketch "Sketch94" against normal blind 10
sketch "Sketch95" plane through (27, 0, 0) normal (1, 0, 0) x (0, 0, -1)
  circle A0 centre (4.7164, 15.5312) radius 2.04
  point P0 (0, 0)
  dimension "d198" = 4.08
  constraints: 1 centre point
  measures "d198" diameter of A0
extrude "Extrusion73" cut sketch "Sketch95" against normal blind 10
body "Solid1"
